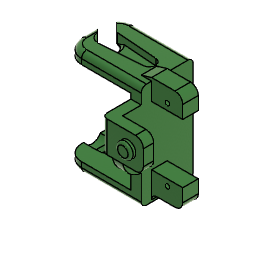
first_joint (Autodesk Fusion 360 design; units mm, degrees)
Autodesk Fusion 360 part; units mm, degrees
sketch "Sketch1" plane through (0, 0, 0) normal (0, 0, 1) x (1, 0, 0)
  line L0 (0, 0) -> (25, 0)
  line L1 (25, 0) -> (25, 20)
  line L2 (25, 20) -> (0, 20)
  line L3 (0, 20) -> (0, 0)
  dimension "d1" = 20
  dimension "d2" = 25
  constraint horizontal L0
  constraint vertical L1
  constraint horizontal L2
  constraint vertical L3
  constraint coincident L0.start L3.end
  measures "d1" distance of L0.start L2.end
  measures "d2" distance of L1.end L2.end
extrude "Extrude1" add sketch "Sketch1" along normal blind 4
sketch "Sketch2" plane through (0, 0, 4) normal (0, 0, 1) x (-1, 0, 0)
  line L0 (0, -20) -> (0, 0)
  line L1 (0, 0) -> (-25, 0)
  line L2 (-25, 0) -> (-25, -20)
  line L3 (-25, -20) -> (0, -20)
  line L4 (-25, 0) -> (-29, 0)
  line L5 (-29, 0) -> (-29, -20)
  line L6 (-29, -20) -> (-25, -20)
  line L7 (-25, -20) -> (-25, 0)
  constraint horizontal L4
  constraint vertical L5
  constraint horizontal L6
  constraint vertical L7
  constraint coincident L1.end L2.start
extrude "Extrude2" add sketch "Sketch2" against normal blind 40.4 contours L2 L4 L5 L6 L7
sketch "Sketch3" plane through (25, 0, 0) normal (-1, 0, 0) x (0, -1, 0)
  line L0 (0, 0) -> (-20, 0)
  line L1 (-20, 0) -> (-20, -36.4)
  line L2 (-20, -36.4) -> (0, -36.4)
  line L3 (0, -36.4) -> (0, 0)
  line L4 (-20, -36.4) -> (0, -36.4)
  line L5 (0, -36.4) -> (0, -32.4)
  line L6 (0, -32.4) -> (-20, -32.4)
  line L7 (-20, -32.4) -> (-20, -36.4)
  dimension "d7" = 4
  constraint horizontal L4
  constraint vertical L5
  constraint horizontal L6
  constraint vertical L7
  constraint coincident L3 L5.end
  constraint coincident L1.end L2.start
  measures "d7" distance of L2.end L5.end
extrude "Extrude3" add sketch "Sketch3" along normal up to surface (25 mm away) contours L1 L2 L3 L4 L5 L6 L7
sketch "Sketch4" plane through (0, 0, 4) normal (0, 0, 1) x (-1, 0, 0)
  line L0 (0, -20) -> (0, 0)
  line L1 (0, 0) -> (-29, 0)
  line L2 (-29, 0) -> (-29, -20)
  line L3 (-29, -20) -> (0, -20)
  line L4 (0, -10) -> (-29, -10) construction
  circle A0 centre (-5.9, -10) radius 3.6
  line L5 (-2.3, -10) -> (-2.3, -15.9675) construction
  circle A1 centre (-22.1, -10) radius 2.4
  line L6 (-22.2778, -12.3934) -> (-6.1667, -13.5901)
  line L7 (-22.2778, -7.6066) -> (-6.1667, -6.4099)
  dimension "d10" = 7.2
  dimension "d11" = 5.9
  dimension "d12" = 4.8
  dimension "d13" = 19.8
  constraint midpoint L0 L4.start
  constraint midpoint L2 L4.end
  constraint coincident L4 A0.centre
  constraint coincident A0 L5.start
  constraint coincident L4 L5.start
  constraint tangent A0 L5
  constraint coincident L4 A1.centre
  constraint coincident A1 L6.start
  constraint coincident A0 L6.end
  constraint tangent A1 L6
  constraint symmetric L4 L6.start L7.start
  constraint symmetric L4 L6.end L7.end
  constraint tangent A0 L7
  measures "d10" diameter of A0
  measures "d11" distance of L0 A0.centre
  measures "d12" diameter of A1
  measures "d13" distance of L5 A1.centre
extrude "Extrude4" cut sketch "Sketch4" along normal mid plane 5 contours A0 | A0 A1 L6 L7 | A1
extrude "Extrude5" cut sketch "Sketch4" against normal blind 9 contours A0
sketch "Sketch5" plane through (0, 0, 0) normal (-1, 0, 0) x (0, -1, 0)
  line L0 (-20, 0) -> (0, 0)
  line L1 (0, 0) -> (0, 4)
  line L2 (0, 4) -> (-20, 4)
  line L3 (-20, 4) -> (-20, 0)
  line L4 (-12.5, 4) -> (-7.5, 4)
  line L5 (-7.5, 4) -> (-7.5, 0)
  line L6 (-7.5, 0) -> (-12.5, 0)
  line L7 (-12.5, 0) -> (-12.5, 4)
  line L8 (-10, 0) -> (-10, 8) construction
  dimension "d19" = 5
  dimension "d20" = 2.5
  constraint horizontal L4
  constraint vertical L5
  constraint horizontal L6
  constraint vertical L7
  constraint coincident L0 L5.end
  constraint coincident L2 L4.start
  constraint midpoint L0 L8.start
  constraint perpendicular L0 L8
  measures "d19" distance of L4.start L4.end
  measures "d20" distance of L5 L8
sketch "Sketch6" plane through (0, 0, -36.4) normal (0, 0, -1) x (1, 0, 0)
  line L0 (0, -20) -> (29, -20)
  line L1 (29, -20) -> (29, 0)
  line L2 (29, 0) -> (0, 0)
  line L3 (0, 0) -> (0, -20)
  line L4 (0, -10) -> (29, -10) construction
  circle A0 centre (5.9, -10) radius 3.15
  dimension "d23" = 6.3
  dimension "d26" = 5.9
  constraint midpoint L3 L4.start
  constraint midpoint L1 L4.end
  constraint coincident L4 A0.centre
  measures "d23" diameter of A0
  measures "d26" distance of L3 A0.centre
extrude "Extrude7" cut sketch "Sketch6" against normal blind 20 contours A0
sketch "Sketch7" plane through (0, 0, 0) normal (-1, 0, 0) x (0, -1, 0)
  line L0 (0, -32.4) -> (-20, -32.4)
  line L1 (-20, -32.4) -> (-20, -36.4)
  line L2 (-20, -36.4) -> (0, -36.4)
  line L3 (0, -36.4) -> (0, -32.4)
  line L4 (-10, -36.4) -> (-10, -32.4) construction
  arc A0 (-13.2, -32.4) -> (-6.8, -32.4) centre (-10, -30.9) ccw
  dimension "d27" = 3.2
  dimension "d28" = 6.4
  dimension "d29" = 1.5
  constraint midpoint L2 L4.start
  constraint midpoint L0 L4.end
  constraint coincident L0 A0.end
  constraint coincident L0 A0.start
  measures "d27" distance of L4.end A0.end
  measures "d28" distance of A0.start A0.end
  measures "d29" distance of L0 A0.centre
extrude "Extrude8" cut sketch "Sketch7" against normal blind 5 contours L0 A0
sketch "Sketch8" plane through (29, 0, 0) normal (1, 0, 0) x (0, 1, 0)
  line L0 (20, 4) -> (0, 4)
  line L1 (0, 4) -> (0, -36.4)
  line L2 (0, -36.4) -> (20, -36.4)
  line L3 (20, -36.4) -> (20, 4)
  line L4 (0, -16.2) -> (20, -16.2) construction
  line L5 (10, 4) -> (10, -36.4) construction
  line L6 (10, 5.2) -> (4, 5.2)
  line L7 (4, 5.2) -> (4, -2.8)
  line L8 (4, -2.8) -> (10, -2.8)
  line L9 (10, -2.8) -> (10, 5.2)
  line L10 (10, -25.6) -> (4, -25.6)
  line L11 (4, -25.6) -> (4, -33.6)
  line L12 (4, -33.6) -> (10, -33.6)
  line L13 (10, -33.6) -> (10, -25.6)
  dimension "d32" = 6
  dimension "d33" = 8
  dimension "d34" = 13.4
  dimension "d70" = 6
  dimension "d71" = 8
  dimension "d72" = 22.8
  constraint midpoint L1 L4.start
  constraint midpoint L3 L4.end
  constraint midpoint L0 L5.start
  constraint midpoint L2 L5.end
  constraint horizontal L6
  constraint vertical L7
  constraint horizontal L8
  constraint vertical L9
  constraint coincident L5 L6.start
  constraint horizontal L10
  constraint vertical L11
  constraint horizontal L12
  constraint vertical L13
  constraint coincident L5 L10.start
  measures "d32" distance of L6.start L6.end
  measures "d33" distance of L6.start L8.end
  measures "d34" distance of L4 L8
  measures "d70" distance of L10.start L10.end
  measures "d71" distance of L10.start L12.end
  measures "d72" distance of L8 L10
extrude "Extrude9" add sketch "Sketch8" along normal blind 12 contours L0 L7 L8 L9 | L0 L6 L7 L9 | L10 L11 L12 L13
sketch "Sketch9" plane through (0, 4, 0) normal (0, -1, 0) x (1, 0, 0)
  line L0 (29, 5.2) -> (29, 4)
  line L1 (41, -2.8) -> (41, 5.2)
  line L2 (41, 5.2) -> (29, 5.2)
  line L3 (35.1, 5.2) -> (35.1, -33) construction
  circle A0 centre (35.1, -0.3) radius 0.85
  line L4 (47.0057, -24.6986) -> (47.0057, -32.7) construction
  line L5 (47.0057, -28.1) -> (42, -28.1) construction
  circle A1 centre (35.1, -28.1) radius 0.85
  line L6 (29, 5.2) -> (25, 4)
  line L7 (29, -32.7) -> (25, -30.6)
  line L8 (25, 4) -> (29, 4)
  line L9 (25, -30.6) -> (29, -30.6)
  line L10 (29, -30.6) -> (29, -32.7)
  line L11 (29, 4) -> (29, -2.8)
  line L12 (29, -2.8) -> (41, -2.8)
  line L13 (29, -25.6) -> (41, -25.6)
  dimension "d37" = 5.9
  dimension "d38" = 1.7
  dimension "d39" = 1.7
  dimension "d78" = 2.5
  dimension "d79" = 2.5
  constraint coincident L2 L3.start
  constraint perpendicular L2 L3
  constraint coincident L3 A0.centre
  constraint vertical L4
  constraint perpendicular L4 L5
  constraint coincident L5 A1.centre
  constraint coincident L3 A1.centre
  constraint coincident L0.start L2.end
  constraint coincident L0.end L8.end
  constraint perpendicular L0 L9
  measures "d37" distance of L1 L3
  measures "d38" diameter of A0
  measures "d39" diameter of A1
  measures "d78" distance of A0.centre L12
  measures "d79" distance of A1.centre L13
extrude "Extrude10" cut sketch "Sketch9" against normal blind 12 contours A0 | A1
extrude "Extrude11" add sketch "Sketch9" against normal up to surface (6 mm away) contours L0 L6 L8 | L7 L9 L10
sketch "Sketch10" plane through (0, 0, 0) normal (0, -1, 0) x (1, 0, 0)
  line L0 (0, 0) -> (25, 0)
  line L1 (25, 0) -> (25, -32.4)
  line L2 (25, -32.4) -> (0, -32.4)
  line L3 (0, -32.4) -> (0, -36.4)
  line L4 (0, -36.4) -> (29, -36.4)
  line L5 (29, 4) -> (0, 4)
  line L6 (0, 4) -> (0, 0)
  line L7 (29, -2) -> (25, -2)
  line L8 (25, -2) -> (25, -24.6991)
  line L9 (25, -24.6991) -> (29, -24.6991)
  line L10 (29, -24.6991) -> (29, -2)
  line L11 (29, -36.4) -> (29, 4)
  constraint horizontal L7
  constraint vertical L8
  constraint horizontal L9
  constraint vertical L10
  constraint coincident L1 L8.end
extrude "Extrude12" add sketch "Sketch10" along normal blind 7.2 contours L1 L7 L8 L9 L10 L11
sketch "Sketch11" plane through (25, 0, 0) normal (-1, 0, 0) x (0, -1, 0)
  line L0 (-20, -32.4) -> (0, -32.4)
  line L1 (0, -32.4) -> (0, -24.6991)
  line L2 (0, -24.6991) -> (7.2, -24.6991)
  line L3 (7.2, -24.6991) -> (7.2, -2)
  line L4 (7.2, -2) -> (0, -2)
  line L5 (0, -2) -> (0, 0)
  line L6 (0, 0) -> (-20, 0)
  line L7 (-20, 0) -> (-20, -32.4)
  line L8 (7.2, -2) -> (11.2, -2)
  line L9 (11.2, -2) -> (11.2, -14)
  line L10 (11.2, -14) -> (7.2, -14)
  line L11 (7.2, -14) -> (7.2, -2)
  dimension "d46" = 4
  dimension "d47" = 12
  constraint horizontal L8
  constraint vertical L9
  constraint horizontal L10
  constraint vertical L11
  constraint coincident L3.end L4.start
  measures "d46" distance of L3.end L8.end
  measures "d47" distance of L3.end L10.end
extrude "Extrude13" add sketch "Sketch11" against normal up to surface (16 mm away) contours L3 L8 L9 L10 L11
sketch "Sketch12" plane through (0, -11.2, 0) normal (0, -1, 0) x (1, 0, 0)
  line L0 (25, -2) -> (25, -14)
  line L1 (25, -14) -> (41, -14)
  line L2 (41, -14) -> (41, -2)
  line L3 (41, -2) -> (25, -2)
  circle A0 centre (35.1, -7.9) radius 3
  dimension "d51" = 6
  dimension "d52" = 5.9
  dimension "d53" = 5.9
  measures "d51" diameter of A0
  measures "d52" distance of L3 A0.centre
  measures "d53" distance of L2 A0.centre
extrude "Extrude14" add sketch "Sketch12" along normal blind 2 contours A0
fillet "Fillet1" radius 1 1 edges at (32.303, -13.2, -8.9848)
fillet "Fillet2" radius 6 4 edges at (0, 20, 2) (0, 0, 2) (0, 0, -34.4) (0, 20, -34.4)
fillet "Fillet4" radius 3 2 edges at (41, -9.2, -2) (41, -9.2, -14)
fillet "Fillet5" radius 8 1 edges at (27, -7.2, -24.6991)
fillet "Fillet6" radius 2 1 edges at (25, -11.2, -8)
fillet "Fillet7" radius 2 11 edges at (17.5, 0, -36.4) (1.7574, 1.7574, -36.4) (0, 10, -36.4) (1.7574, 18.2426, -36.4) (17.5, 20, -36.4) (0, 10, 4) (1.7574, 1.7574, 4) (17.5, 0, 4) (17.5, 20, 4) (1.7574, 18.2426, 4) (0, 10, 4)
extrude "Extrude15" cut 1 faces at (18.0185, 10, 1.5) along direction (0, 0, 1) blind 17
chamfer "Chamfer1" distance 1 angle 45 1 edges at (9.5, 10, 1.5)
fillet "Fillet8" radius 3 2 edges at (41, 7, 5.2) (41, 7, -33.6)
fillet "Fillet9" radius 2 1 edges at (29, 7, -33.6)
sketch "Sketch14" plane through (0, 0, 4) normal (0, 0, 1) x (-1, 0, 0)
  line L0 (-6, -2) -> (-29, -2)
  line L1 (-29, -2) -> (-29, -4)
  line L2 (-29, -4) -> (-25, -4)
  line L3 (-25, -4) -> (-25, -10)
  line L4 (-25, -10) -> (-29, -10)
  line L5 (-29, -10) -> (-29, -18)
  line L6 (-29, -18) -> (-6, -18)
  arc A0 (-6, -18) -> (-2, -14) centre (-6, -14) ccw
  line L7 (-2, -14) -> (-2, -6)
  arc A1 (-2, -6) -> (-6, -2) centre (-6, -6) ccw
  arc A2 (-6.1667, -13.5901) -> (-6.1667, -6.4099) centre (-5.9, -10) ccw
  line L8 (-6.1667, -13.5901) -> (-22.2778, -12.3934)
  arc A3 (-22.2778, -7.6066) -> (-22.2778, -12.3934) centre (-22.1, -10) ccw
  line L9 (-22.2778, -7.6066) -> (-6.1667, -6.4099)
  line L10 (-5.9, -10) -> (5.3752, -21.2752) construction
  line L11 (-5.9, -10) -> (10.0456, -10) construction
  line L12 (-5.9778, -13.5992) -> (6.2826, -25.8595)
  line L13 (-2.3008, -9.9222) -> (9.9595, -22.1826)
  line L14 (0, -19.577) -> (3.677, -15.9)
  line L15 (-2.3008, -9.9222) -> (-3.7524, -8.4706)
  line L16 (-3.7524, -8.4706) -> (-7.6661, -12.3844)
  line L17 (-5.9778, -13.5992) -> (-7.4294, -12.1476)
  dimension "d85" = 45
  dimension "d86" = 2.6
  dimension "d87" = -5.2
  constraint horizontal L11
  constraint coincident A2.centre L10.start
  constraint coincident A2 L12.start
  constraint parallel L10 L12
  constraint coincident L12 L14.start
  constraint coincident L13 L14.end
  constraint perpendicular L13 L14
  constraint parallel L13 L15
  constraint perpendicular L15 L16
  constraint coincident L16 L17.end
  constraint perpendicular L16 L17
  measures "d85" angle of L10 L11
  measures "d86" distance of L10 L12
extrude "Extrude17" cut sketch "Sketch14" against normal blind 8 contours A0 L7 L12 L13 L14 | A0 L7 A2 L12 L13 | A2 L15 L16 L17
equation "d5 = -34.6 mm - 2.4 mm - 3 mm - 0.4 mm"
equation "d13 = 16.2 mm + ( ( 7.2 / 2 ) * 1 mm )"
equation "d34 = ( 22.8 / 2 ) * 1 mm + 2 mm"
equation "d72 = ( 11.4 * 2 ) * 1 mm"
